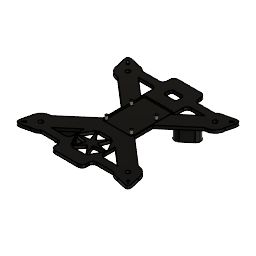
ICARUS 3 POLEGADAS CHASSI (Autodesk Fusion 360 design; units mm, degrees)
Autodesk Fusion 360 part; units mm, degrees
sketch "Esboço1" plane through (0, 0, 0) normal (0, 0, 1) x (1, 0, 0)
  line L0 (14, -75) -> (-14, -75)
  line L1 (-19, -70) -> (-19, 70)
  line L2 (-14, 75) -> (14, 75)
  line L3 (19, 70) -> (19, -70)
  line L4 (19, -75) -> (-19, 75) construction
  line L5 (-19, -75) -> (19, 75) construction
  arc A0 (-14, 75) -> (-19, 70) centre (-14, 70) ccw
  arc A1 (19, 70) -> (14, 75) centre (14, 70) ccw
  arc A2 (14, -75) -> (19, -70) centre (14, -70) ccw
  arc A3 (-19, -70) -> (-14, -75) centre (-14, -70) ccw
  dimension "d1" = 38
  dimension "d2" = 150
  dimension "d3" = 5
  dimension "d4" = 5
  dimension "d5" = 5
  dimension "d6" = 5
  constraint horizontal L0
  constraint perpendicular L0 L1
  constraint parallel L0 L2
  constraint parallel L1 L3
  constraint coincident L4 origin
  constraint coincident L5 origin
  constraint coincident L4.end L2
  constraint coincident L4.end L1
  constraint tangent L2 A0
  constraint tangent L1 A0
  constraint coincident L5.end L2
  constraint coincident L5.end L3
  constraint tangent L2 A1
  constraint tangent L3 A1
  constraint coincident L4.start L0
  constraint coincident L4.start L3
  constraint tangent L0 A2
  constraint tangent L3 A2
  constraint coincident L5.start L0
  constraint coincident L5.start L1
  constraint tangent L0 A3
  constraint tangent L1 A3
  measures "d1" distance of L4.end L5.end
  measures "d2" distance of L5.start L4.end
  measures "d3" radius of A0
  measures "d4" radius of A1
  measures "d5" radius of A2
  measures "d6" radius of A3
extrude "Extrusão1" add sketch "Esboço1" along normal blind 3.5 makes body 1
sketch "Esboço2" plane through (0, 0, 3.5) normal (0, 0, 1) x (-1, 0, 0)
  arc A0 (14, -75) -> (19, -70) centre (14, -70) ccw
  line L0 (19, -70) -> (19, 70)
  arc A1 (19, 70) -> (14, 75) centre (14, 70) ccw
  line L1 (14, 75) -> (-14, 75)
  arc A2 (-14, 75) -> (-19, 70) centre (-14, 70) ccw
  line L2 (-19, 70) -> (-19, -70)
  arc A3 (-19, -70) -> (-14, -75) centre (-14, -70) ccw
  line L3 (-14, -75) -> (14, -75)
  line L4 (19, 0) -> (-19, 0) construction
  line L5 (16, 13.75) -> (-16, 13.75)
  line L6 (-18, 11.75) -> (-18, -35.75)
  line L7 (-16, -37.75) -> (16, -37.75)
  line L8 (18, -35.75) -> (18, 11.75)
  arc A4 (-16, 13.75) -> (-18, 11.75) centre (-16, 11.75) ccw
  arc A5 (18, 11.75) -> (16, 13.75) centre (16, 11.75) ccw
  arc A6 (16, -37.75) -> (18, -35.75) centre (16, -35.75) ccw
  arc A7 (-18, -35.75) -> (-16, -37.75) centre (-16, -35.75) ccw
  line L9 (17.5355, -73.5355) -> (17.4142, -37.1642) construction
  line L10 (-17.5355, -73.5355) -> (-17.5355, -37.1642) construction
  line L11 (17.5355, -73.5355) -> (-17.5355, -73.5355) construction
  line L12 (17.4142, -37.1642) -> (-17.5355, -37.1642) construction
  line L13 (0, -73.5355) -> (0, -37.75) construction
  line L14 (-5, -50.6428) -> (5, -50.6428)
  line L15 (7.5, -53.1428) -> (7.5, -58.1428)
  line L16 (5, -60.6428) -> (-5, -60.6428)
  line L17 (-7.5, -58.1428) -> (-7.5, -53.1428)
  line L18 (-7.5, -50.6428) -> (7.5, -60.6428) construction
  line L19 (7.5, -50.6428) -> (-7.5, -60.6428) construction
  arc A8 (5, -60.6428) -> (7.5, -58.1428) centre (5, -58.1428) ccw
  arc A9 (-7.5, -58.1428) -> (-5, -60.6428) centre (-5, -58.1428) ccw
  arc A10 (7.5, -53.1428) -> (5, -50.6428) centre (5, -53.1428) ccw
  arc A11 (-5, -50.6428) -> (-7.5, -53.1428) centre (-5, -53.1428) ccw
  line L20 (0, 13.75) -> (0, -37.75)
  line L21 (18, 11.75) -> (18, 13.75) construction
  line L22 (18, 13.75) -> (16, 13.75) construction
  line L23 (18, 13.75) -> (-18.0566, 13.75) construction
  line L24 (-18.0566, 13.75) -> (-18, 11.75) construction
  line L25 (18, 13.75) -> (-18, 13.75)
  line L26 (-18, 13.75) -> (-18, -22.25)
  line L27 (-18, -22.25) -> (18, -22.25)
  line L28 (18, -22.25) -> (18, 13.75)
  line L29 (0, -22.25) -> (0, 13.75)
  line L30 (0, -4.25) -> (18, -4.25) construction
  line L31 (-15.25, 11) -> (15.25, 11) construction
  line L32 (15.25, 11) -> (15.25, -19.5) construction
  line L33 (15.25, -19.5) -> (-15.25, -19.5) construction
  line L34 (-15.25, -19.5) -> (-15.25, 11) construction
  line L35 (-15.25, 11) -> (15.25, -19.5) construction
  line L36 (15.25, 11) -> (-15.25, -19.5) construction
  circle A12 centre (15.25, -19.5) radius 1.375
  circle A13 centre (15.25, 11) radius 1.375
  circle A14 centre (-15.25, 11) radius 1.375
  circle A15 centre (-15.25, -19.5) radius 1.375
  line L37 (0, 75) -> (0, 13.75) construction
  line L38 (0, 44.375) -> (19, 44.375) construction
  line L39 (0, 44.375) -> (-19, 44.375) construction
  line L40 (9.5, 27.9205) -> (9.5, 44.375) construction
  line L41 (9.5, 44.375) -> (9.5, 60.8295) construction
  line L42 (-9.5, 27.9205) -> (-9.5, 44.375) construction
  line L43 (-9.5, 44.375) -> (-9.5, 60.8295) construction
  line L44 (0, 44.375) -> (0, 34.875)
  line L45 (8.1768, 29.5507) -> (0.7764, 38.6684)
  line L46 (-0.7764, 38.6684) -> (-8.1768, 29.5507)
  arc A16 (0.7764, 38.6684) -> (-0.7764, 38.6684) centre (0, 38.0382) ccw
  line L47 (7.4004, 27.9205) -> (-7.4004, 27.9205)
  arc A17 (7.4004, 27.9205) -> (8.1768, 29.5507) centre (7.4004, 28.9205) ccw
  arc A18 (-8.1768, 29.5507) -> (-7.4004, 27.9205) centre (-7.4004, 28.9205) ccw
  line L48 (16.9266, 44.0442) -> (5.3303, 42.1941)
  arc A19 (17.9502, 42.5567) -> (16.9266, 44.0442) centre (17.0842, 43.0567) ccw
  line L49 (17.9502, 42.5567) -> (10.5498, 29.7388)
  arc A20 (8.7498, 29.8815) -> (10.5498, 29.7388) centre (9.6838, 30.2388) ccw
  line L50 (4.5538, 40.8493) -> (8.7498, 29.8815)
  arc A21 (5.3303, 42.1941) -> (4.5538, 40.8493) centre (5.4878, 41.2066) ccw
  line L51 (8.7498, 58.8685) -> (4.5538, 47.9007)
  arc A22 (10.5498, 59.0112) -> (8.7498, 58.8685) centre (9.6838, 58.5112) ccw
  line L52 (10.5498, 59.0112) -> (17.9502, 46.1933)
  arc A23 (16.9266, 44.7058) -> (17.9502, 46.1933) centre (17.0842, 45.6933) ccw
  line L53 (5.3303, 46.5559) -> (16.9266, 44.7058)
  arc A24 (4.5538, 47.9007) -> (5.3303, 46.5559) centre (5.4878, 47.5434) ccw
  line L54 (-8.1768, 59.1993) -> (-0.7764, 50.0816)
  arc A25 (-7.4004, 60.8295) -> (-8.1768, 59.1993) centre (-7.4004, 59.8295) ccw
  line L55 (-7.4004, 60.8295) -> (7.4004, 60.8295)
  arc A26 (8.1768, 59.1993) -> (7.4004, 60.8295) centre (7.4004, 59.8295) ccw
  line L56 (0.7764, 50.0816) -> (8.1768, 59.1993)
  arc A27 (-0.7764, 50.0816) -> (0.7764, 50.0816) centre (0, 50.7118) ccw
  line L57 (-16.9266, 44.7058) -> (-5.3303, 46.5559)
  arc A28 (-17.9502, 46.1933) -> (-16.9266, 44.7058) centre (-17.0842, 45.6933) ccw
  line L58 (-17.9502, 46.1933) -> (-10.5498, 59.0112)
  arc A29 (-8.7498, 58.8685) -> (-10.5498, 59.0112) centre (-9.6838, 58.5112) ccw
  line L59 (-4.5538, 47.9007) -> (-8.7498, 58.8685)
  arc A30 (-5.3303, 46.5559) -> (-4.5538, 47.9007) centre (-5.4878, 47.5434) ccw
  line L60 (-8.7498, 29.8815) -> (-4.5538, 40.8493)
  arc A31 (-10.5498, 29.7388) -> (-8.7498, 29.8815) centre (-9.6838, 30.2388) ccw
  line L61 (-10.5498, 29.7388) -> (-17.9502, 42.5567)
  arc A32 (-16.9266, 44.0442) -> (-17.9502, 42.5567) centre (-17.0842, 43.0567) ccw
  line L62 (-5.3303, 42.1941) -> (-16.9266, 44.0442)
  arc A33 (-4.5538, 40.8493) -> (-5.3303, 42.1941) centre (-5.4878, 41.2066) ccw
  point P0 (0, -55.6428)
  point P1 (0, -4.25)
  dimension "d74" = 2
  dimension "d75" = 2
  dimension "d76" = 2
  dimension "d79" = 15
  dimension "d80" = 10
  dimension "d81" = 2.5
  dimension "d82" = 2.5
  dimension "d83" = 2.5
  dimension "d84" = 2.5
  dimension "d87" = 36
  dimension "d88" = 36
  dimension "d89" = 30.5
  dimension "d90" = 30.5
  dimension "d91" = 2.75
  dimension "d93" = 360
  dimension "d102" = 1
  dimension "d103" = 1
  dimension "d104" = 1
  constraint midpoint L0 L4.start
  constraint midpoint L2 L4.end
  constraint horizontal L5
  constraint perpendicular L5 L6
  constraint parallel L5 L7
  constraint parallel L6 L8
  constraint tangent L5 A4
  constraint tangent L6 A4
  constraint tangent L8 A5
  constraint tangent L5 A5
  constraint tangent L7 A6
  constraint tangent L8 A6
  constraint equal A5 A6
  constraint tangent L7 A7
  constraint tangent L6 A7
  constraint midpoint A0 L9.start
  constraint midpoint A6 L9.end
  constraint midpoint A3 L10.start
  constraint parallel L2 L10
  constraint perpendicular L10 L12
  constraint midpoint L11 L13.start
  constraint midpoint L7 L13.end
  constraint perpendicular L7 L13
  constraint horizontal L14
  constraint perpendicular L14 L15
  constraint parallel L14 L16
  constraint parallel L15 L17
  constraint coincident L18 P0
  constraint coincident L19 P0
  constraint midpoint L13 P0
  constraint coincident L18.end L15
  constraint coincident L18.end L16
  constraint tangent L15 A8
  constraint tangent L16 A8
  constraint coincident L19.end L16
  constraint coincident L19.end L17
  constraint tangent L16 A9
  constraint tangent L17 A9
  constraint coincident L19.start L14
  constraint coincident L19.start L15
  constraint tangent L14 A10
  constraint tangent L15 A10
  constraint coincident L18.start L14
  constraint coincident L18.start L17
  constraint tangent L14 A11
  constraint tangent L17 A11
  constraint midpoint L5 L20.start
  constraint tangent A5 L21
  constraint tangent A5 L22
  constraint perpendicular L2 L23
  constraint horizontal L25
  constraint vertical L26
  constraint horizontal L27
  constraint vertical L28
  constraint midpoint L27 L29.start
  constraint perpendicular L23 L29
  constraint midpoint L29 P1
  constraint midpoint L28 L30.end
  constraint horizontal L31
  constraint perpendicular L31 L32
  constraint parallel L31 L33
  constraint parallel L32 L34
  constraint coincident L35 P1
  constraint coincident L36 P1
  constraint coincident P1 L30.start
  constraint coincident L32.end L33.start
  constraint midpoint L1 L37.start
  constraint midpoint L37 L38.start
  constraint coincident L0 L38.end
  constraint perpendicular L0 L38
  constraint coincident L2 L39.end
  constraint perpendicular L2 L39
  constraint midpoint L38 L40.end
  constraint perpendicular L38 L40
  constraint perpendicular L38 L41
  constraint symmetric L37 L40.start L42.start
  constraint symmetric L37 L40.end L42.end
  constraint symmetric L37 L41.end L43.end
  constraint tangent L45 A16
  constraint tangent L46 A16
  constraint coincident L40.start L45
  constraint coincident L40.start L47
  constraint tangent L45 A17
  constraint tangent L47 A17
  constraint coincident L42.start L47
  constraint coincident L42.start L46
  constraint tangent L47 A18
  constraint tangent L46 A18
  measures "d74" radius of A4
  measures "d75" radius of A5
  measures "d76" radius of A7
  measures "d79" distance of L18.end L19.end
  measures "d80" distance of L19.start L18.end
  measures "d81" radius of A8
  measures "d82" radius of A9
  measures "d83" radius of A10
  measures "d84" radius of A11
  measures "d87" distance of L21.end L25.end
  measures "d88" distance of L21.end L27.end
  measures "d89" distance of L32.end L33.end
  measures "d90" distance of L31.end L32.end
  measures "d91" diameter of A12
  measures "d102" radius of A16
  measures "d103" radius of A17
  measures "d104" radius of A18
extrude "Extrusão2" cut sketch "Esboço2" against normal blind 2 contours L5 L8 A5 L20 L25 L27 L28 L29 | L5 L6 A4 L20 L25 L26 L27 L29 | L7 L8 A6 L20 L27 | L6 L7 A7 L20 L27 | A12 | A13 | A14 | A15 bodies 1
sketch "Esboço3" plane through (0, 0, 3.5) normal (0, 0, 1) x (-1, 0, 0)
  line L0 (-16, 13.75) -> (16, 13.75)
  line L1 (18, 11.75) -> (18, -35.75)
  line L2 (16, -37.75) -> (-16, -37.75)
  line L3 (-18, -35.75) -> (-18, 11.75)
  arc A0 (14, -75) -> (19, -70) centre (14, -70) ccw
  line L4 (19, -70) -> (19, 70)
  arc A1 (19, 70) -> (14, 75) centre (14, 70) ccw
  line L5 (14, 75) -> (-14, 75)
  arc A2 (-14, 75) -> (-19, 70) centre (-14, 70) ccw
  line L6 (-19, 70) -> (-19, -70)
  arc A3 (-19, -70) -> (-14, -75) centre (-14, -70) ccw
  line L7 (-14, -75) -> (14, -75)
  line L8 (19, 0) -> (19, -11.25) construction
  line L9 (19, 0) -> (19.7942, 11.2219) construction
  line L10 (19, -11.25) -> (-19, -11.25) construction
  line L11 (19.7942, 11.2219) -> (-19, 11.2219) construction
  line L12 (-1.8732, 1.767) -> (0, 0) construction
  line L13 (-53.1, 53.1) -> (53.1, 53.1) construction
  line L14 (53.1, 53.1) -> (53.1, -53.1) construction
  line L15 (53.1, -53.1) -> (-53.1, -53.1) construction
  line L16 (-53.1, -53.1) -> (-53.1, 53.1) construction
  line L17 (-53.1, 53.1) -> (53.1, -53.1) construction
  line L18 (53.1, 53.1) -> (-53.1, -53.1) construction
  circle A4 centre (53.1, -53.1) radius 12.5
  circle A5 centre (-53.1, -53.1) radius 12.5
  circle A6 centre (-53.1, 53.1) radius 12.5
  circle A7 centre (53.1, 53.1) radius 12.5
  line L19 (53.1, -40.6) -> (19, -11.25)
  line L20 (19, -11.25) -> (19, -70) construction
  line L21 (39.6446, -53.1) -> (40.6, -53.1) construction
  line L22 (40.6, -53.1) -> (19, -34.5088)
  line L23 (82.0691, 0) -> (-103.2974, 0) construction
  line L24 (0, -65.516) -> (0, 69.07) construction
  line L25 (40.6, 53.1) -> (19, 34.5088)
  line L26 (53.1, 40.6) -> (19, 11.25)
  line L27 (-53.1, -40.6) -> (-19, -11.25)
  line L28 (-39.6446, -53.1) -> (-40.6, -53.1) construction
  line L29 (-40.6, -53.1) -> (-19, -34.5088)
  line L30 (-53.1, 40.6) -> (-19, 11.25)
  line L31 (-40.6, 53.1) -> (-19, 34.5088)
  spline S0 degree 2 poles (65.6, -53.0754) (70.6231, -70.6231) (52.8232, -65.5969) knots 0 0 0 2.969399 2.969399 2.969399 weights 1 2.821651 1
  spline S1 degree 2 poles (62.2524, -59.9872) (66.3064, -66.2499) (60.2708, -62.2226) knots 0 0 0 1.233128 1.233128 1.233128 weights 1 4.892995 1
  line L32 (62.8537, -60.9176) -> (61.0529, -62.7437) construction
  arc A8 (62.2524, -59.9872) -> (60.2708, -62.2226) centre (61.2616, -61.1049) ccw
  circle A9 centre (53.1, -53.1) radius 2.5
  arc A10 (-60.2708, -62.2226) -> (-62.2524, -59.9872) centre (-61.2616, -61.1049) ccw
  spline S2 degree 2 poles (-62.2524, -59.9872) (-66.3064, -66.2499) (-60.2708, -62.2226) knots 0 0 0 1.233128 1.233128 1.233128 weights 1 4.892995 1
  spline S3 degree 2 poles (-65.6, -53.0754) (-70.6231, -70.6231) (-52.8232, -65.5969) knots 0 0 0 2.969399 2.969399 2.969399 weights 1 2.821651 1
  circle A11 centre (-53.1, -53.1) radius 2.5
  spline S4 degree 2 poles (65.6, 53.0754) (70.6231, 70.6231) (52.8232, 65.5969) knots 0 0 0 2.969399 2.969399 2.969399 weights 1 2.821651 1
  spline S5 degree 2 poles (62.2524, 59.9872) (66.3064, 66.2499) (60.2708, 62.2226) knots 0 0 0 1.233128 1.233128 1.233128 weights 1 4.892995 1
  arc A12 (60.2708, 62.2226) -> (62.2524, 59.9872) centre (61.2616, 61.1049) ccw
  circle A13 centre (53.1, 53.1) radius 2.5
  circle A14 centre (-53.1, 53.1) radius 2.5
  spline S6 degree 2 poles (-62.2524, 59.9872) (-66.3064, 66.2499) (-60.2708, 62.2226) knots 0 0 0 1.233128 1.233128 1.233128 weights 1 4.892995 1
  arc A15 (-62.2524, 59.9872) -> (-60.2708, 62.2226) centre (-61.2616, 61.1049) ccw
  spline S7 degree 2 poles (-65.6, 53.0754) (-70.6231, 70.6231) (-52.8232, 65.5969) knots 0 0 0 2.969399 2.969399 2.969399 weights 1 2.821651 1
  arc A16 (-18, -35.75) -> (-16, -37.75) centre (-16, -35.75) ccw
  arc A17 (-16, 13.75) -> (-18, 11.75) centre (-16, 11.75) ccw
  arc A18 (18, 11.75) -> (16, 13.75) centre (16, 11.75) ccw
  arc A19 (16, -37.75) -> (18, -35.75) centre (16, -35.75) ccw
  line L33 (19, -34.5088) -> (19, -11.25) construction
  point P0 (31.554, -34.8832)
  dimension "d13" = 11.25
  dimension "d14" = 11.25
  dimension "d41" = 106.2
  dimension "d42" = 106.2
  dimension "d43" = 25
  dimension "d44" = 25
  dimension "d45" = 25
  dimension "d46" = 25
  dimension "d67" = 5
  constraint midpoint L4 L8.start
  constraint coincident L6 L10.end
  constraint perpendicular L6 L10
  constraint coincident L6 L11.end
  constraint perpendicular L6 L11
  constraint coincident L12.end origin
  constraint horizontal L13
  constraint perpendicular L13 L14
  constraint parallel L13 L15
  constraint parallel L14 L16
  constraint coincident L17 L12.end
  constraint coincident L18 L12.end
  constraint coincident L14.end L15.start
  constraint coincident L15.end L16.start
  constraint coincident L13.start L16.end
  constraint coincident L13.end L14.start
  constraint coincident A4 L19.start
  constraint coincident L14 L19.start
  constraint coincident A0.end L4.start
  constraint tangent A0 L20
  constraint coincident L15 L21.start
  constraint coincident A4 L21.end
  constraint coincident L15 L21.end
  constraint coincident L20 L22.end
  constraint parallel L19 L22
  constraint perpendicular L1 L23
  constraint perpendicular L23 L24
  constraint symmetric L8.end L23 L26.end
  constraint symmetric L19.start L23 L26.start
  constraint symmetric L21.end L23 L25.start
  constraint symmetric L22.end L23 L25.end
  constraint symmetric L8.end L24 L10.end
  constraint symmetric L19.start L24 L27.start
  constraint symmetric L21.start L24 L28.start
  constraint symmetric L21.end L24 L28.end
  constraint symmetric L22.end L24 L29.end
  constraint symmetric L24 L25.start L31.start
  constraint symmetric L24 L25.end L31.end
  constraint symmetric L24 L26.start L30.start
  constraint symmetric L24 L26.end L30.end
  constraint coincident A4 S0.end
  constraint coincident A4 S0.start
  constraint coincident S1 L32.start
  constraint coincident A4 L32.start
  constraint coincident S1 L32.end
  constraint coincident A4 L32.end
  constraint concentric A4 A9
  constraint symmetric L24 S0.end S3.end
  constraint symmetric L24 S0.start S3.start
  constraint symmetric L24 S0 S3
  constraint symmetric L24 S1.start A10.end
  constraint symmetric L24 S1.end A10.start
  constraint symmetric L24 S1 S2
  constraint symmetric L24 A8 A10
  constraint symmetric L24 A9 A11
  constraint symmetric L23 S0.end S4.end
  constraint symmetric L23 S0.start S4.start
  constraint symmetric L23 S0 S4
  constraint symmetric L23 S1.start S5.start
  constraint symmetric L23 S1.end S5.end
  constraint symmetric L23 S1 S5
  constraint symmetric L23 A8 A12
  constraint symmetric L23 A9 A13
  constraint symmetric L23 A10.end S6.start
  constraint symmetric L23 A10.start S6.end
  constraint symmetric L23 A10 A15
  constraint symmetric L23 S2 S6
  constraint symmetric L23 S3.start S7.start
  constraint symmetric L23 S3.end S7.end
  constraint symmetric L23 S3 S7
  constraint symmetric L23 A11 A14
  measures "d13" distance of L8.start L8.end
  measures "d14" distance of L8.start L9.end
  measures "d41" distance of L14.end L15.end
  measures "d42" distance of L13.end L14.end
  measures "d43" diameter of A4
  measures "d44" diameter of A5
  measures "d45" diameter of A6
  measures "d46" diameter of A7
  measures "d67" diameter of A9
extrude "Extrusão3" add sketch "Esboço3" against normal blind 3.5 contours L4 A4 L19 L22 | A4 S1 A8 | L6 A5 L27 L29 | L4 A7 L25 L26 | A4 S0 S1 | A5 A10 S2 | A7 S5 A12 | L6 A6 L30 L31 | A5 S2 S3 | A7 S4 S5 | A6 S6 A15 | A5 A10 S2 | A6 S6 S7 | A7 S5 A12 | A6 S6 A15 picked at (56.5902, -60.5787) bodies 1
sketch "Esboço4" plane through (0, 0, 0) normal (0, 0, -1) x (1, 0, 0)
  arc A0 (-19, -70) -> (-14, -75) centre (-14, -70) ccw
  line L0 (-14, -75) -> (14, -75)
  arc A1 (14, -75) -> (19, -70) centre (14, -70) ccw
  line L1 (19, -70) -> (19, -34.5088)
  arc A2 (19, 70) -> (14, 75) centre (14, 70) ccw
  line L2 (14, 75) -> (-14, 75)
  arc A3 (-14, 75) -> (-19, 70) centre (-14, 70) ccw
  line L3 (-19, 70) -> (-19, 34.5088)
  line L4 (19, 0) -> (-19, 0) construction
  line L5 (53.1, -40.6) -> (40.6, -53.1) construction
  line L6 (23.957, -38.7753) -> (40.6, -53.1) construction
  line L7 (19, -11.25) -> (19, -34.5088) construction
  line L8 (19, -11.25) -> (53.1, -40.6) construction
  line L9 (0, -75) -> (0, 75) construction
  line L10 (53.1, 0) -> (-49.7297, 0) construction
  line L11 (19, 11.25) -> (53.1, 40.6) construction
  line L12 (53.1, 40.6) -> (40.6, 53.1) construction
  line L13 (23.957, 38.7753) -> (40.6, 53.1) construction
  line L14 (19, 11.25) -> (19, 34.5088) construction
  line L15 (-19, 11.25) -> (-19, 34.5088) construction
  line L16 (-23.957, 38.7753) -> (-40.6, 53.1) construction
  line L17 (-19, 11.25) -> (-53.1, 40.6) construction
  line L18 (-53.1, 40.6) -> (-40.6, 53.1) construction
  line L19 (-19, -11.25) -> (-53.1, -40.6) construction
  line L20 (-53.1, -40.6) -> (-40.6, -53.1) construction
  line L21 (-23.957, -38.7753) -> (-40.6, -53.1) construction
  line L22 (-19, -11.25) -> (-19, -34.5088) construction
  line L23 (29.8, -43.8044) -> (41.2998, -30.4435) construction
  line L24 (36.05, -25.925) -> (24.5502, -39.2859) construction
  line L25 (35.5499, -37.124) -> (30.3001, -32.6054) construction
  line L26 (19, -22.8794) -> (46.85, -46.85) construction
  line L27 (44.6888, -37.124) -> (34.1892, -28.0869)
  arc A4 (34.1892, -28.0869) -> (26.411, -37.124) centre (30.3001, -32.6054) ccw
  line L28 (26.411, -37.124) -> (36.9106, -46.161)
  arc A5 (36.9106, -46.161) -> (44.6888, -37.124) centre (40.7997, -41.6425) ccw
  line L29 (40.7997, -41.6425) -> (30.3001, -32.6054) construction
  arc A6 (-44.6888, -37.124) -> (-36.9106, -46.161) centre (-40.7997, -41.6425) ccw
  line L30 (-26.411, -37.124) -> (-36.9106, -46.161)
  arc A7 (-26.411, -37.124) -> (-34.1892, -28.0869) centre (-30.3001, -32.6054) ccw
  line L31 (-44.6888, -37.124) -> (-34.1892, -28.0869)
  line L32 (26.411, 37.124) -> (36.9106, 46.161)
  arc A8 (44.6888, 37.124) -> (36.9106, 46.161) centre (40.7997, 41.6425) ccw
  line L33 (44.6888, 37.124) -> (34.1892, 28.0869)
  arc A9 (26.411, 37.124) -> (34.1892, 28.0869) centre (30.3001, 32.6054) ccw
  line L34 (-26.411, 37.124) -> (-36.9106, 46.161)
  arc A10 (-34.1892, 28.0869) -> (-26.411, 37.124) centre (-30.3001, 32.6054) ccw
  line L35 (-44.6888, 37.124) -> (-34.1892, 28.0869)
  arc A11 (-36.9106, 46.161) -> (-44.6888, 37.124) centre (-40.7997, 41.6425) ccw
  circle A12 centre (53.1, 53.1) radius 2.5
  spline S0 degree 2 poles (61.0529, 62.7437) (66.272, 66.216) (62.8537, 60.9176) knots -1.214656 -1.214656 -1.214656 -0.021592 -0.021592 -0.021592 weights 1.114883 4.768557 1.133943
  arc A13 (62.8537, 60.9176) -> (61.0529, 62.7437) centre (53.1, 53.1) ccw
  spline S1 degree 2 poles (-62.8537, 60.9176) (-66.272, 66.216) (-61.0529, 62.7437) knots 0.021592 0.021592 0.021592 1.214656 1.214656 1.214656 weights 1.133943 4.768557 1.114883
  arc A14 (-61.0529, 62.7437) -> (-62.8537, 60.9176) centre (-53.1, 53.1) ccw
  circle A15 centre (-53.1, 53.1) radius 2.5
  circle A16 centre (53.1, -53.1) radius 2.5
  spline S2 degree 2 poles (62.8537, -60.9176) (66.272, -66.216) (61.0529, -62.7437) knots 0.021592 0.021592 0.021592 1.214656 1.214656 1.214656 weights 1.133943 4.768557 1.114883
  arc A17 (61.0529, -62.7437) -> (62.8537, -60.9176) centre (53.1, -53.1) ccw
  circle A18 centre (-53.1, -53.1) radius 2.5
  arc A19 (-60.2708, -62.2226) -> (-62.2524, -59.9872) centre (-61.2616, -61.1049) ccw
  spline S3 degree 2 poles (-60.2708, -62.2226) (-66.3064, -66.2499) (-62.2524, -59.9872) knots -1.233128 -1.233128 -1.233128 0 0 0 weights 1 4.892995 1
  line L36 (19, -34.5088) -> (40.6, -53.1)
  arc A20 (40.6, -53.1) -> (52.8232, -65.5969) centre (53.1, -53.1) ccw
  spline S4 degree 2 poles (52.8232, -65.5969) (70.6231, -70.6231) (65.6, -53.0754) knots -2.969399 -2.969399 -2.969399 0 0 0 weights 1 2.821651 1
  arc A21 (65.6, -53.0754) -> (53.1, -40.6) centre (53.1, -53.1) ccw
  line L37 (53.1, -40.6) -> (19, -11.25)
  line L38 (19, -11.25) -> (19, 11.25)
  line L39 (19, 11.25) -> (53.1, 40.6)
  arc A22 (53.1, 40.6) -> (65.6, 53.0754) centre (53.1, 53.1) ccw
  spline S5 degree 2 poles (65.6, 53.0754) (70.6231, 70.6231) (52.8232, 65.5969) knots 0 0 0 2.969399 2.969399 2.969399 weights 1 2.821651 1
  arc A23 (52.8232, 65.5969) -> (40.6, 53.1) centre (53.1, 53.1) ccw
  line L40 (40.6, 53.1) -> (19, 34.5088)
  line L41 (19, 34.5088) -> (19, 70)
  line L42 (-19, 34.5088) -> (-40.6, 53.1)
  arc A24 (-40.6, 53.1) -> (-52.8232, 65.5969) centre (-53.1, 53.1) ccw
  spline S6 degree 2 poles (-52.8232, 65.5969) (-70.6231, 70.6231) (-65.6, 53.0754) knots -2.969399 -2.969399 -2.969399 0 0 0 weights 1 2.821651 1
  arc A25 (-65.6, 53.0754) -> (-53.1, 40.6) centre (-53.1, 53.1) ccw
  line L43 (-53.1, 40.6) -> (-19, 11.25)
  line L44 (-19, 11.25) -> (-19, -11.25)
  line L45 (-19, -11.25) -> (-53.1, -40.6)
  arc A26 (-53.1, -40.6) -> (-65.6, -53.0754) centre (-53.1, -53.1) ccw
  spline S7 degree 2 poles (-65.6, -53.0754) (-70.6231, -70.6231) (-52.8232, -65.5969) knots 0 0 0 2.969399 2.969399 2.969399 weights 1 2.821651 1
  arc A27 (-52.8232, -65.5969) -> (-40.6, -53.1) centre (-53.1, -53.1) ccw
  line L46 (-40.6, -53.1) -> (-19, -34.5088)
  line L47 (-19, -34.5088) -> (-19, -70)
  line L48 (-40.6, -53.1) -> (-24, -53.1)
  line L49 (24, -53.1) -> (40.6, -53.1)
  line L50 (-44.1638, -61.8404) -> (-24, -61.8404)
  line L51 (24, -61.8404) -> (44.1638, -61.8404)
  line L52 (24, 61.8404) -> (44.1638, 61.8404)
  line L53 (24, 53.1) -> (40.6, 53.1)
  line L54 (-44.1638, 61.8404) -> (-24, 61.8404)
  line L55 (-40.6, 53.1) -> (-24, 53.1)
  line L56 (19, 0) -> (-19, 0) construction
  line L57 (19, 41.0491) -> (19, 48.1)
  arc A28 (24, 53.1) -> (19, 48.1) centre (24, 48.1) ccw
  line L58 (19, 66.8404) -> (19, 70)
  arc A29 (19, 66.8404) -> (24, 61.8404) centre (24, 66.8404) ccw
  arc A30 (19, 41.0491) -> (23.957, 38.7753) centre (22, 41.0491) ccw
  line L59 (-19, 48.1) -> (-19, 41.0491)
  arc A31 (-23.957, 38.7753) -> (-19, 41.0491) centre (-22, 41.0491) ccw
  arc A32 (-19, 48.1) -> (-24, 53.1) centre (-24, 48.1) ccw
  line L60 (-19, 66.8404) -> (-19, 70)
  arc A33 (-24, 61.8404) -> (-19, 66.8404) centre (-24, 66.8404) ccw
  line L61 (-19, -70) -> (-19, -66.8404)
  arc A34 (-19, -66.8404) -> (-24, -61.8404) centre (-24, -66.8404) ccw
  line L62 (19, -66.8404) -> (19, -73.5355)
  arc A35 (24, -61.8404) -> (19, -66.8404) centre (24, -66.8404) ccw
  line L63 (19, -41.0491) -> (19, -48.1)
  arc A36 (23.957, -38.7753) -> (19, -41.0491) centre (22, -41.0491) ccw
  line L64 (-19, -48.1) -> (-19, -41.0491)
  arc A37 (-19, -41.0491) -> (-23.957, -38.7753) centre (-22, -41.0491) ccw
  arc A38 (-24, -53.1) -> (-19, -48.1) centre (-24, -48.1) ccw
  arc A39 (19, -48.1) -> (24, -53.1) centre (24, -48.1) ccw
  point P0 (35.5499, -37.124)
  dimension "d109" = 5
  dimension "d110" = 5
  dimension "d111" = 3
  dimension "d112" = 3
  dimension "d113" = 5
  dimension "d114" = 5
  dimension "d115" = 5
  dimension "d116" = 5
  dimension "d117" = 3
  dimension "d118" = 3
  dimension "d119" = 5
  dimension "d120" = 5
  constraint coincident L1.end L7.end
  constraint midpoint L0 L9.start
  constraint midpoint L2 L9.end
  constraint symmetric L5.start L10 L11.end
  constraint symmetric L5.end L10 L12.end
  constraint symmetric L1.end L10 L14.end
  constraint symmetric L7.start L10 L11.start
  constraint symmetric L5.start L9 L19.end
  constraint symmetric L5.end L9 L20.end
  constraint symmetric L1.end L9 L22.end
  constraint symmetric L7.start L9 L19.start
  constraint symmetric L9 L11.start L15.start
  constraint symmetric L9 L11.end L17.end
  constraint symmetric L9 L12.end L16.end
  constraint symmetric L9 L14.end L3.end
  constraint coincident L8 L23.end
  constraint perpendicular L8 L23
  constraint midpoint L8 L24.start
  constraint coincident L6 L24.end
  constraint perpendicular L6 L24
  constraint midpoint L23 P0
  constraint midpoint L24 L25.end
  constraint midpoint L7 L26.start
  constraint midpoint L5 L26.end
  constraint tangent L27 A4
  constraint tangent A4 L28
  constraint parallel L27 L28
  constraint tangent L28 A5
  constraint tangent L27 A5
  constraint coincident L25.end A4.centre
  constraint perpendicular L24 L29
  constraint coincident P0 L25.start
  constraint midpoint L29 P0
  constraint symmetric L9 L27.start A6.start
  constraint symmetric L9 L27.end A7.end
  constraint symmetric L9 A4.end L30.start
  constraint symmetric L9 L28.end A6.end
  constraint symmetric L9 A4 A7
  constraint symmetric L9 A5 A6
  constraint symmetric L10 L27.start A8.start
  constraint symmetric L10 L27.end L33.end
  constraint symmetric L10 A4.end L32.start
  constraint symmetric L10 L28.end L32.end
  constraint symmetric L10 A4 A9
  constraint symmetric L10 A5 A8
  constraint symmetric L10 A6.end L34.end
  constraint symmetric L10 A6.start L35.start
  constraint symmetric L10 A6 A11
  constraint symmetric L10 L30.start L34.start
  constraint symmetric L10 A7.end A10.start
  constraint symmetric L10 A7 A10
  constraint coincident L20.end L21.end
  constraint perpendicular L47 L48
  constraint coincident L5.end L6.end
  constraint perpendicular L1 L49
  constraint midpoint A27 L50.start
  constraint perpendicular L47 L50
  constraint midpoint A20 L51.end
  constraint perpendicular L1 L51
  constraint symmetric L4.start L10 L56.start
  constraint symmetric L4.end L10 L56.end
  constraint symmetric L10 L20.end L16.end
  constraint symmetric L10 L5.end L12.end
  constraint symmetric L10 L50.start L54.start
  constraint symmetric L10 L51.end L52.end
  constraint tangent L53 A28
  constraint tangent L57 A28
  constraint coincident A2.start L41.end
  constraint tangent L52 A29
  constraint tangent L58 A29
  constraint coincident L14.end L13
  constraint tangent L57 A30
  constraint tangent L13 A30
  constraint tangent L16 A31
  constraint tangent L59 A31
  constraint tangent L55 A32
  constraint tangent L59 A32
  constraint coincident A3.end L3.start
  constraint tangent L54 A33
  constraint tangent L60 A33
  constraint coincident A0.start L47.end
  constraint tangent L50 A34
  constraint tangent L61 A34
  constraint perpendicular L51 L62
  constraint tangent L51 A35
  constraint tangent L62 A35
  constraint coincident L6 L23.start
  constraint coincident L1.end L6
  constraint tangent L6 A36
  constraint tangent L63 A36
  constraint coincident L22.end L21
  constraint tangent L64 A37
  constraint tangent L21 A37
  constraint tangent L48 A38
  constraint tangent L64 A38
  constraint tangent L63 A39
  constraint tangent L49 A39
  measures "d109" radius of A28
  measures "d110" radius of A29
  measures "d111" radius of A30
  measures "d112" radius of A31
  measures "d113" radius of A32
  measures "d114" radius of A33
  measures "d115" radius of A34
  measures "d116" radius of A35
  measures "d117" radius of A36
  measures "d118" radius of A37
  measures "d119" radius of A38
  measures "d120" radius of A39
extrude "Extrusão4" add sketch "Esboço4" along normal blind 15 contours L27 A4 L28 A5 | A6 L30 A7 L31 | L32 A8 L33 A9 | L34 A10 L35 A11 bodies 1
extrude "Extrusão5" cut sketch "Esboço2" against normal blind 4 contours L14 L15 L16 L17 A8 A9 A10 A11 bodies 1
extrude "Extrusão6" add sketch "Esboço2" along normal blind 5 separate body contours A12 | A13 | A14 | A15 makes body 2 at (13.8767, 19.5685, 6.8333) makes body 3 at (13.8767, -10.9315, 6.8333) makes body 4 at (-16.6233, 19.5685, 6.8333) makes body 5 at (-16.6233, -10.9315, 6.8333)
extrude "Extrusão7" add sketch "Esboço4" against normal blind 3.5 contours A27 L47 L48 L50 A34 A38 | L1 A20 L49 L51 A35 A39 bodies 1
extrude "Extrusão8" add sketch "Esboço4" against normal blind 3.5 contours L3 A24 L54 L55 A32 A33 | A23 L41 L52 L53 A28 A29 bodies 1
extrude "Extrusão9" cut sketch "Esboço2" against normal blind 4 contours L45 L46 A16 L47 A17 A18 | L48 A19 L49 A20 L50 A21 | L51 A22 L52 A23 L53 A24 | L54 A25 L55 A26 L56 A27 | L57 A28 L58 A29 L59 A30 | L60 A31 L61 A32 L62 A33 bodies 1
equation "d64 = 0.738333"
equation "d66 = 0.830307"
equation "d68 = d66"
equation "d69 = d64"
equation "d70 = d64"
equation "d71 = d66"
equation "d72 = d68"
equation "d73 = d69"
